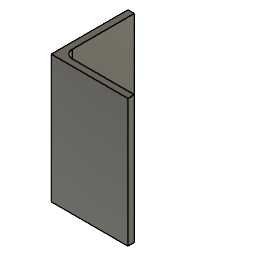
L-60×60×5 (Autodesk Fusion 360 design; units mm, degrees)
Autodesk Fusion 360 part; units mm, degrees
note: some values were not read from the file. Set by a fixed rule: which sketch regions a step uses.
sketch "スケッチ1" plane through (0, 0, 0) normal (0, 0, 1) x (1, 0, 0)
  line L0 (0, 60) -> (0, 0)
  line L1 (60, 0) -> (60, 5)
  line L2 (0, 0) -> (60, 0)
  line L3 (60, 5) -> (11.5, 5)
  line L4 (5, 11.5) -> (5, 60)
  arc A0 (5, 11.5) -> (11.5, 5) centre (11.5, 11.5) ccw
  line L5 (5, 60) -> (0, 60)
extrude "押し出し1" add sketch "スケッチ1" along normal blind 100
